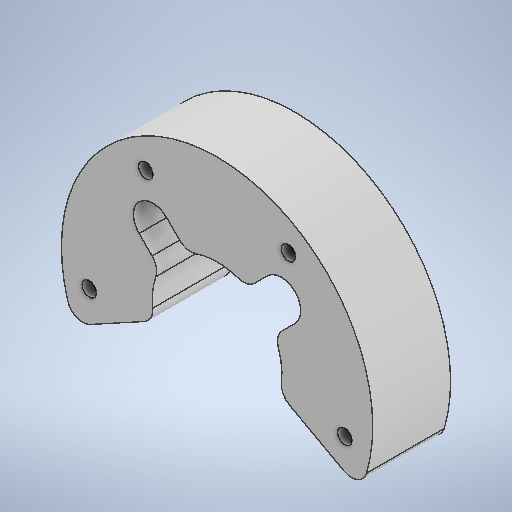
# Autodesk Inventor part: RT_ARM_MC_008_Capstand_Support
Saved by Autodesk Inventor 2025.3 (Build 293356000, 356)
## iProperties
Created: 2026-07-28
Part Number: RT_ARM_MC_008_Capstand_Support
Material: Generic
Document SubType Name: Modeling
Designer: louis
Density: 1 g/cm^3
Appearance: Default
Author: louis
Autodesk Inventor part; units mm, degrees
ref_plane "YZ Plane" through (0, 0, 0) normal (1, 0, 0) x (0, 1, 0)
ref_plane "XZ Plane" through (0, 0, 0) normal (0, 1, 0) x (-1, 0, 0)
ref_plane "XY Plane" through (0, 0, 0) normal (0, 0, 1) x (1, 0, 0)
sketch "Sketch1" plane through (0, 0, 0) normal (0, 0, 1) x (1, 0, 0)
  circle A0 centre (0, 0) radius 60
  circle A1 centre (0, -84) radius 72 construction
  circle A2 centre (0, 0) radius 12 construction
  line L0 (0, -84) -> (0, 0) construction
  line L1 (0, 0) -> (0, 60) construction
  circle A3 centre (0, 0) radius 35 construction
  circle A4 centre (0, 0) radius 50 construction
  line L2 (-50.3895, -32.5714) -> (-8.3983, 8.5714) construction
  line L3 (8.3983, 8.5714) -> (50.3895, -32.5714) construction
  circle A5 centre (0, 0) radius 25
  circle A6 centre (0, 0) radius 60
  line L4 (-50.3895, -32.5714) -> (-24.0638, -6.7776)
  line L5 (24.0638, -6.7776) -> (50.3895, -32.5714)
  circle A7 centre (-24.7487, 24.7487) radius 7.5
  circle A8 centre (24.7487, 24.7487) radius 7.5
  line L6 (-24.7487, 24.7487) -> (24.7487, 24.7487) construction
  circle A9 centre (-24.7487, -24.7487) radius 7.5 construction
  circle A10 centre (24.7487, -24.7487) radius 7.5 construction
  line L7 (-24.7487, 24.7487) -> (-24.7487, -24.7487) construction
  line L8 (24.7487, -24.7487) -> (24.7487, 24.7487) construction
  line L9 (24.7487, -24.7487) -> (-24.7487, -24.7487) construction
  line L10 (-30.052, 19.4454) -> (-22.1667, 11.5601)
  line L11 (-19.4454, 30.052) -> (-11.5601, 22.1667)
  line L12 (19.4454, 30.052) -> (11.5601, 22.1667)
  line L13 (30.052, 19.4454) -> (22.1667, 11.5601)
  line L14 (-49.2404, -8.6824) -> (0, 0) construction
  line L15 (-55.0993, -23.75) -> (-24.0638, -6.7776)
  line L16 (24.0638, -6.7776) -> (55.0993, -23.75)
  point P0 (-27.4754, 41.7744)
  point P1 (27.4754, 41.7744)
  point P2 (49.2404, -8.6824)
  dimension "d0" = 120
  dimension "d4" = 100
  dimension "d1" = 144
  dimension "d2" = 24
  dimension "d3" = 70
  dimension "d5" = 50
  dimension "d6" = 15
  dimension "d7" = 15
  dimension "d8" = 15
  dimension "d9" = 15
  dimension "d10" = 45
  dimension "d11" = 45
  dimension "d12" = 100
  dimension "d15" = 200
  dimension "d30" = 10
  dimension "d32" = 10
  constraints: 34 end point, 22 point on circle, 9 centre point, 9 tangent, 7 coincident, 3 perpendicular, 2 parallel, 2 point on line, 1 collinear, 1 horizontal, 1 vertical, 11 other
  measures "d1" diameter of A1
  measures "d2" diameter of A2
  measures "d3" diameter of A3
  measures "d5" diameter of A5
  measures "d6" diameter of A7
  measures "d7" diameter of A8
  measures "d8" diameter of A9
  measures "d9" diameter of A10
  measures "d10" angle of L6 L12
  measures "d11" angle of L11 L6
  measures "d12" angle of L14 L1
  measures "d30" distance of L15.start L4.start
  measures "d32" distance of L16.end L3.end
extrude "Extrusion1" add sketch "Sketch1" along normal blind 30 contours A0 L16 A5 L13 A8 L12 L11 A7 L10 L15
fillet "Fillet1" radius 6 8 edges at (24.0638, -6.7776, 15) (-24.0638, -6.7776, 15) (-22.1667, 11.5601, 15) (-11.5601, 22.1667, 15) (11.5601, 22.1667, 15) (22.1667, 11.5601, 15) (-55.0993, -23.75, 15) (55.0993, -23.75, 15)
hole "Hole1" at (-49.2404, -8.6824, 0) at (-27.4754, 41.7744, 0) at (27.4754, 41.7744, 0) at (49.2404, -8.6824, 0) direction (0, 0, 1) diameter 5.6 end through all
body "Solid1"
